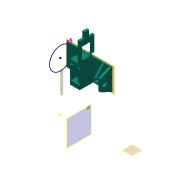
# Autodesk Inventor part: 30_Cube_XYZ_Stage_micrometer
Saved by Autodesk Inventor 2019 (Build 230136000, 136)
## iProperties
Created: 2020-01-27
Part Number: 30_Cube_XYZ_Stage_micrometer
Material: Generic
Document SubType Name: Modeling
Designer: diederichbenedict
Density: 1 g/cm^3
Appearance: IPHT_Türkis
Author: diederichbenedict
Autodesk Inventor part; units mm, degrees
ref_plane "Work Plane1" through (-87, 111.025, -16.9) normal (0, 0, 1) x (0, -1, 0)
ref_plane "Work Plane2" through (-77.1, 158.7453, 0.9792) normal (-1, 0, 0) x (0, 0, 1)
sketch "Sketch2" plane through (-77.1, 158.7453, 0.9792) normal (-1, 0, 0) x (0, 0, 1)
  circle A0 centre (-3.6792, 33.2797) radius 0.9 projected
  circle A1 centre (12.0208, -13.4394) radius 0.9 projected
  circle A2 centre (-14.9792, -12.5703) radius 0.9 projected
  line L0 (4.6208, 1.0297) -> (4.6208, 8.2797) projected
  line L1 (-4.8792, 8.2797) -> (-4.8792, 1.0297) projected
  line L2 (-4.8792, 1.0297) -> (4.6208, 1.0297) projected
  line L3 (4.6208, 8.2797) -> (-4.8792, 8.2797) projected
  line L4 (15.3208, -8.9703) -> (15.3208, 6.4797) projected
  line L5 (-5.6792, 35.2797) -> (3.4208, 35.2797) projected
  line L6 (20.1208, 22.4797) -> (4.1208, 22.4797) projected
  line L7 (-22.6852, 20.4797) -> (-8.6792, 20.4797) projected
  line L8 (15.3208, 6.4797) -> (15.3208, 22.4797)
  line L9 (15.3208, 22.4797) -> (4.1208, 22.4797)
  line L10 (4.1208, 22.4797) -> (4.1208, 35.2797)
  line L11 (4.1208, 35.2797) -> (-5.6792, 35.2797)
  line L12 (-16.3292, -14.4703) -> (-17.9792, -12.8203) projected
  line L13 (-16.3292, -14.4703) -> (-11.8329, -14.4703)
  line L14 (-11.8329, -14.4703) -> (-11.8329, -22.4688)
  line L15 (-11.8329, -22.4688) -> (15.3208, -22.4688)
  line L16 (15.3208, -22.4688) -> (15.3208, 6.4797)
  line L17 (9.9041, -17.695) -> (9.9041, 9.5842)
  line L18 (9.9041, 9.5842) -> (-12.605, 9.5842)
  line L19 (-12.605, 9.5842) -> (-12.605, -12.6165)
  line L20 (-12.605, -12.6165) -> (-10.7484, -12.6165)
  line L21 (-10.7484, -12.6165) -> (-5.6698, -17.695)
  line L22 (-5.6698, -17.695) -> (9.9041, -17.695)
  line L23 (-16.3292, -14.4703) -> (-17.8792, -12.9203)
  line L24 (-5.6792, 35.2797) -> (-5.6792, 20.4797)
  line L25 (-5.6792, 20.4797) -> (-17.8792, 20.4797)
  line L26 (-17.8792, -12.9203) -> (-17.8792, 20.4797)
  point P0 (-0.9792, -158.7453)
  constraints: 36 end point, 8 perpendicular, 3 collinear, 3 parallel, 3 vertical, 2 point on line, 1 horizontal
extrude "Extrusion1" add sketch "Sketch2" along normal blind 5 contours L16 L15 L14 L13 L12 L26 L7 L25 L24 L5 L11 L10 L6 L8 L4
sketch "Sketch3" plane through (-77.1, 158.7453, 0.9792) normal (1, 0, 0) x (0, -1, 0)
  circle A0 centre (-33.2797, 3.6792) radius 0.9 projected
  circle A1 centre (12.5703, 14.9792) radius 0.9 projected
  circle A2 centre (13.4394, -12.0208) radius 0.9 projected
  circle A3 centre (-33.2797, 3.6792) radius 2
  line L0 (-35.2797, -4.1208) -> (-35.2797, 5.6792) projected
  line L1 (14.4703, 16.3292) -> (14.4703, 11.8329) projected
  circle A4 centre (13.4394, -12.0208) radius 0.9 projected
  circle A5 centre (13.4394, -12.0208) radius 2
  circle A6 centre (12.5703, 14.9792) radius 1.9509
  point P0 (158.7453, 0.9792)
  dimension "d2" = 4
  constraints: 3 centre point, 3 coincident, 1 tangent
  measures "d2" diameter of A5
ref_plane "Work Plane6" through (-30.75, 17.2, 24.2) normal (0, -1, 0) x (1, 0, 0)
ref_plane "Work Plane8" through (-30.75, 12.2, 24.2) normal (0, -1, 0) x (1, 0, 0)
ref_plane "Work Plane3" through (-75, 13.4, 4.2) normal (0, -1, 0) x (1, 0, 0)
ref_plane "Work Plane7" through (-75, 18.4, 4.2) normal (0, -1, 0) x (1, 0, 0)
ref_plane "Work Plane9" through (-75, 13.4, 4.2) normal (0, -1, 0) x (1, 0, 0)
ref_plane "Work Plane4" through (-87, 111.025, -16.9) normal (0, 0, 1) x (0, -1, 0)
sketch "Sketch5" plane through (-87, 111.025, -16.9) normal (0, 0, 1) x (0, -1, 0)
  line L0 (-16.9, -46.4) -> (-16.9, -41.9) projected
  line L1 (-16.9, -41.9) -> (-21.4, -41.9) projected
  line L2 (-21.4, 41.9) -> (-21.4, -41.9) projected
  line L3 (-21.4, 41.9) -> (-16.9, 41.9) projected
  line L4 (-16.9, 41.9) -> (-16.9, 46.4) projected
  line L5 (-16.9, 46.4) -> (16.9, 46.4) projected
  line L6 (16.9, 46.4) -> (16.9, 41.9) projected
  line L7 (16.9, 41.9) -> (21.4, 41.9) projected
  line L8 (21.4, -41.9) -> (21.4, 41.9) projected
  line L9 (21.4, -41.9) -> (16.9, -41.9) projected
  line L10 (16.9, -41.9) -> (16.9, -46.4) projected
  line L11 (16.9, -46.4) -> (-16.9, -46.4) projected
  circle A0 centre (-19.9, 44.9) radius 1.45 projected
  circle A1 centre (-19.9, -44.9) radius 1.45 projected
  circle A2 centre (19.9, -44.9) radius 1.45 projected
  circle A3 centre (19.9, 44.9) radius 1.45 projected
  line L12 (-24.9, 47.9) -> (-24.9, -47.9) projected
  arc A4 (-24.9, -47.9) -> (-22.9, -49.9) centre (-22.9, -47.9) ccw projected
  line L13 (-22.9, -49.9) -> (22.9, -49.9) projected
  arc A5 (22.9, -49.9) -> (24.9, -47.9) centre (22.9, -47.9) ccw projected
  line L14 (24.9, -47.9) -> (24.9, 47.9) projected
  arc A6 (24.9, 47.9) -> (22.9, 49.9) centre (22.9, 47.9) ccw projected
  line L15 (22.9, 49.9) -> (-22.9, 49.9) projected
  arc A7 (-22.9, 49.9) -> (-24.9, 47.9) centre (-22.9, 47.9) ccw projected
  line L16 (-25.2515, 9.9) -> (-70.2, 9.9) projected
  line L17 (-24.9, 9.9) -> (24.9, 9.9)
  arc A8 (-19.2018, -3.8292) -> (-18.9105, -6.1599) centre (-19.9, -5.1) ccw
  arc A9 (-18.9105, 6.1599) -> (-19.2018, 3.8292) centre (-19.9, 5.1) ccw
  arc A10 (18.9105, -6.1599) -> (19.2018, -3.8292) centre (19.9, -5.1) ccw
  arc A11 (19.2018, 3.8292) -> (18.9105, 6.1599) centre (19.9, 5.1) ccw
  circle A12 centre (-19.9, -5.1) radius 1.45
  circle A13 centre (-19.9, 5.1) radius 1.45
  circle A14 centre (19.9, 5.1) radius 1.45
  circle A15 centre (19.9, -5.1) radius 1.45
  point P0 (111.025, 87)
  point P1 (-21.4, 9.9)
  point P2 (21.4, 9.9)
  constraints: 8 centre point, 8 point on circle, 7 point on line, 4 coincident, 4 concentric, 2 end point, 1 perpendicular, 16 other
ref_plane "Work Plane5" through (-136.9, 88.125, -16.9) normal (-1, 0, 0) x (0, 1, 0)
sketch "Sketch6" plane through (-136.9, 88.125, -16.9) normal (-1, 0, 0) x (0, 1, 0)
  line L0 (47.8, 0) -> (47.8, 6) projected
  line L1 (-2, 0) -> (-2, 6) projected
  line L2 (42.8, 8) -> (3, 8) projected
  circle A0 centre (22.9, -16.9) radius 24.9
  point P0 (-88.125, -16.9)
  constraints: 3 tangent, 1 centre point
extrude "Extrusion4" add sketch "Sketch5" along normal blind 3
sketch "Sketch7" plane through (-77.1, 181.225, 16.3) normal (0, 0, 1) x (0, -1, 0)
  line L0 (44.9485, 0) -> (0, 0) projected
  line L1 (0, 0) -> (0, -5) projected
  line L2 (44.9485, -5) -> (0, -5) projected
  line L3 (44.9485, 0) -> (44.9485, -5) projected
  circle A0 centre (90.1, -54.8) radius 1.45 projected
  circle A1 centre (50.3, -54.8) radius 1.45 projected
  line L4 (45.3, 38) -> (45.3, -57.8) projected
  arc A2 (45.3, -57.8) -> (47.3, -59.8) centre (47.3, -57.8) ccw projected
  line L5 (47.3, -59.8) -> (93.1, -59.8) projected
  arc A3 (93.1, -59.8) -> (95.1, -57.8) centre (93.1, -57.8) ccw projected
  line L6 (95.1, -57.8) -> (95.1, 38) projected
  line L7 (54.9485, 0) -> (54.9485, -0.5)
  line L8 (45.3, 38) -> (45.3, -57.8) projected
  line L9 (45.3, -5) -> (44.9485, -5)
  line L10 (54.9485, -22.1938) -> (54.9485, -21.6938)
  line L11 (54.9485, 0) -> (83.0578, 0)
  line L12 (83.0578, 0) -> (83.0578, -5)
  line L13 (83.0578, -5) -> (54.9485, -5)
  line L14 (54.9485, -5) -> (54.9485, 0)
  line L15 (54.9485, -22.1938) -> (83.0578, -22.1938)
  line L16 (83.0578, -22.1938) -> (83.0578, -17.1938)
  line L17 (83.0578, -17.1938) -> (54.9485, -17.1938)
  line L18 (54.9485, -17.1938) -> (54.9485, -22.1938)
  line L19 (83.0578, -22.1938) -> (86.0578, -22.1938)
  line L20 (86.0578, -22.1938) -> (86.0578, -21.6938)
  line L21 (86.0578, -21.6938) -> (83.0578, -21.6938)
  line L22 (83.0578, -21.6938) -> (83.0578, -22.1938)
  line L23 (83.0578, 0) -> (86.0578, 0)
  line L24 (86.0578, 0) -> (86.0578, -0.5)
  line L25 (86.0578, -0.5) -> (83.0578, -0.5)
  line L26 (83.0578, -0.5) -> (83.0578, 0)
  line L27 (95.1, -57.8) -> (95.1, 38) projected
  line L28 (86.0578, 0) -> (95.1, 0)
  line L29 (95.1, 0) -> (95.1, -22.1938)
  line L30 (95.1, -22.1938) -> (86.0578, -22.1938)
  line L31 (86.0578, -22.1938) -> (86.0578, 0)
  arc A4 (95.1, 38) -> (93.1, 40) centre (93.1, 38) ccw projected
  line L32 (93.1, 40) -> (47.3, 40) projected
  arc A5 (47.3, 40) -> (45.3, 38) centre (47.3, 38) ccw projected
  line L33 (44.9485, 0) -> (51.9485, 0)
  line L34 (51.9485, 0) -> (51.9485, -22.1938)
  line L35 (51.9485, -22.1938) -> (44.9485, -22.1938)
  line L36 (44.9485, -22.1938) -> (44.9485, 0)
  line L37 (51.9485, 0) -> (54.9485, 0)
  line L38 (54.9485, 0) -> (54.9485, -0.5)
  line L39 (54.9485, -0.5) -> (51.9485, -0.5)
  line L40 (51.9485, -0.5) -> (51.9485, 0)
  line L41 (51.9485, -22.1938) -> (54.9485, -22.1938)
  line L42 (54.9485, -22.1938) -> (54.9485, -21.6938)
  line L43 (54.9485, -21.6938) -> (51.9485, -21.6938)
  line L44 (51.9485, -21.6938) -> (51.9485, -22.1938)
  point P0 (181.225, 77.1)
  point P1 (37.3, 0)
  dimension "d10" = 0.5
  dimension "d12" = 0.5
  dimension "d13" = 5
  dimension "d14" = 3
  dimension "d15" = 0.5
  dimension "d37" = 3
  dimension "d40" = 7
  dimension "d41" = 3
  dimension "d42" = 0.5
  dimension "d43" = 3
  dimension "d44" = 0.5
  constraints: 70 end point, 16 parallel, 9 horizontal, 8 perpendicular, 6 point on line, 2 other
  measures "d10" distance of L7.start L7.end
  measures "d12" distance of L10.start L10.end
  measures "d13" distance of L16.end L15.end
  measures "d14" distance of L21.end L20.end
  measures "d15" distance of L20.end L19.end
  measures "d37" distance between parallel lines of L31 L12
  measures "d40" distance of L34.end L35.end
  measures "d41" distance of L38.end L39.end
  measures "d42" distance of L37.end L38.end
  measures "d43" distance of L43.end L42.end
  measures "d44" distance of L42.end L10.start
extrude "Extrusion5" add sketch "Sketch7" against normal blind 29 contours L33 L4 L9 L3 | L9 L4 L35 L36 | L33 L34 L35 L4 | L37 L7 L39 L34 | L11 L12 L13 L14 L7 | L34 L43 L10 L41 | L23 L24 L25 L12 | L10 L18 L17 L16 L15 | L28 L6 L30 L20 L31 L24 | L16 L21 L20 L19
sketch "Sketch8" plane through (-77.1, 181.225, -12.7) normal (0, 0, -1) x (0, 1, 0)
  line L0 (-95.1, 0) -> (-95.1, -22.1938) projected
  line L1 (-54.9485, -21.6938) -> (-54.9485, -17.1938) projected
  line L2 (-54.9485, -17.1938) -> (-83.0578, -17.1938) projected
  line L3 (-83.0578, -17.1938) -> (-83.0578, -21.6938) projected
  line L4 (-83.0578, -21.6938) -> (-86.0578, -21.6938) projected
  line L5 (-86.0578, -21.6938) -> (-86.0578, -0.5) projected
  line L6 (-86.0578, -0.5) -> (-83.0578, -0.5) projected
  line L7 (-83.0578, -0.5) -> (-83.0578, -5) projected
  line L8 (-83.0578, -5) -> (-54.9485, -5) projected
  line L9 (-54.9485, -5) -> (-54.9485, -0.5) projected
  line L10 (-44.9485, 0) -> (-95.1, 0) projected
  line L11 (-95.1, -22.1938) -> (-44.9485, -22.1938) projected
  line L12 (-44.9485, -22.1938) -> (-44.9485, 0) projected
  line L13 (-51.9485, -0.5) -> (-51.9485, -21.6938) projected
  line L14 (-51.9485, -21.6938) -> (-54.9485, -21.6938) projected
  line L15 (-54.9485, -0.5) -> (-51.9485, -0.5) projected
  line L16 (-95.1, -22.1938) -> (-86.0578, -22.1938)
  line L17 (-86.0578, -22.1938) -> (-86.0578, 0)
  line L18 (-86.0578, 0) -> (-95.1, 0)
  line L19 (-95.1, 0) -> (-95.1, -22.1938)
  constraints: 8 end point, 2 parallel, 1 horizontal, 1 perpendicular, 1 point on line
extrude "Extrusion6" add sketch "Sketch8" along normal up to surface (1.2 mm away) contours L10 L17 L5 L11 L0
sketch "Sketch9" plane through (-87, 111.025, -16.9) normal (0, 0, -1) x (0, 1, 0)
  circle A0 centre (-19.9, -5.1) radius 1.45 projected
  circle A1 centre (-19.9, 5.1) radius 1.45 projected
  point P0 (-111.025, 87)
extrude "Extrusion7" add sketch "Sketch9" against normal up to surface (33.2 mm away)
sketch "Sketch10" plane through (-37.1, 133.925, -16.9) normal (1, 0, 0) x (0, -1, 0)
  circle A0 centre (22.9, -16.9) radius 6.335 projected
  line L0 (35.4, -2.4) -> (35.4, -26.4) construction
  line L1 (35.4, -26.4) -> (10.4, -26.4) construction
  line L2 (10.4, -26.4) -> (10.4, -2.4) construction
  line L3 (10.4, -2.4) -> (35.4, -2.4) construction
  circle A1 centre (12.4, -4.4) radius 1.05 construction
  circle A2 centre (12.4, -16.9) radius 1.05 construction
  circle A3 centre (33.4, -16.9) radius 1.05 construction
  circle A4 centre (33.4, -4.4) radius 1.05 construction
  line L4 (17.4, -8) -> (14.4, -8) construction
  line L5 (17.4, -6) -> (17.4, -8) construction
  line L6 (14.4, -6) -> (17.4, -6) construction
  line L7 (14.4, -8) -> (14.4, -6) construction
  line L8 (47.8, 0) -> (47.8, 6) construction
  line L9 (-2, 0) -> (-2, 6) construction
  line L10 (47.8, 0) -> (35.4, -26.4)
  line L11 (35.4, -26.4) -> (10.4, -26.4)
  line L12 (10.4, -26.4) -> (-2, 0)
  line L13 (-2, 0) -> (47.8, 0)
  circle A5 centre (33.4, -4.4) radius 1.05 projected
  circle A6 centre (33.4, -16.9) radius 1.05 projected
  circle A7 centre (12.4, -4.4) radius 1.05 projected
  circle A8 centre (12.4, -16.9) radius 1.05 projected
  circle A9 centre (33.4, -4.4) radius 0.75
  circle A10 centre (33.4, -16.9) radius 0.75
  circle A11 centre (12.4, -4.4) radius 0.75
  circle A12 centre (12.4, -16.9) radius 0.75
  point P0 (133.925, -16.9)
  dimension "d45" = 1.5
  dimension "d46" = 1.5
  dimension "d47" = 1.5
  dimension "d48" = 1.5
  constraints: 8 end point, 4 centre point, 4 coincident, 1 collinear, 1 perpendicular
  measures "d45" diameter of A9
  measures "d46" diameter of A10
  measures "d47" diameter of A11
  measures "d48" diameter of A12
extrude "Extrusion8" add sketch "Sketch10" against normal blind 5 contours L10 L11 L12 L13
sketch "Sketch15" plane through (-42.1, 133.925, -16.9) normal (-1, 0, 0) x (0, -1, 0)
  circle A0 centre (33.4, 4.4) radius 1.05 projected
  circle A1 centre (33.4, 16.9) radius 1.05 projected
  circle A2 centre (12.4, 4.4) radius 1.05 projected
  circle A3 centre (12.4, 16.9) radius 1.05 projected
  line L0 (35.398, 2.4813) -> (31.4341, 2.4813)
  line L1 (31.4341, 2.4813) -> (31.4341, 18.8854)
  line L2 (31.4341, 18.8854) -> (35.398, 18.8854)
  line L3 (35.398, 18.8854) -> (35.398, 2.4813)
  line L4 (10.368, 2.4813) -> (14.0327, 2.4813)
  line L5 (14.0327, 2.4813) -> (14.0327, 18.5364)
  line L6 (14.0327, 18.5364) -> (10.368, 18.5364)
  line L7 (10.368, 18.5364) -> (10.368, 2.4813)
  point P0 (133.925, 16.9)
  constraints: 16 end point, 4 parallel, 2 horizontal, 2 perpendicular, 1 point on line
ref_plane "Work Plane14" through (8, -4.95, -16.9) normal (0, 1, 0) x (-1, 0, 0)
ref_plane "Work Plane15" through (-4.5, 41.5, 2.4) normal (0, 1, 0) x (0, 0, 1)
ref_plane "Work Plane19" through (-45.5, 98.525, -14.5) normal (1, 0, 0) x (0, 1, 0)
extrude "Extrusion16" add sketch "Sketch15" along normal up to surface (3.4 mm away)
sketch "Sketch18" plane through (-87, 111.025, -13.9) normal (0, 0, 1) x (0, -1, 0)
  line L0 (12.5, 40.6) -> (-12.5, 40.6) projected
  line L1 (12.5, 40.6) -> (-12.5, 40.6) projected
  line L2 (12.5, 41.5) -> (12.5, 40.6) projected
  line L3 (12.5, 41.5) -> (10.4, 41.5) projected
  line L4 (10.4, 43.9) -> (10.4, 41.5) projected
  line L5 (-10.4, 43.9) -> (10.4, 43.9) projected
  line L6 (-10.4, 43.9) -> (-10.4, 41.5) projected
  line L7 (-10.4, 41.5) -> (-12.5, 41.5) projected
  line L8 (-12.5, 41.5) -> (-12.5, 40.6) projected
  line L9 (8, 42.7) -> (8, 43.1) projected
  line L10 (-8, 42.7) -> (8, 42.7) projected
  line L11 (-8, 43.1) -> (-8, 42.7) projected
  line L12 (8, 43.1) -> (-8, 43.1) projected
  line L13 (-12.9725, 39.4492) -> (13.4306, 39.4492)
  line L14 (13.4306, 39.4492) -> (13.4306, 41.5)
  line L15 (13.4306, 41.5) -> (-12.9725, 41.5)
  line L16 (-12.9725, 41.5) -> (-12.9725, 39.4492)
  point P0 (111.025, 87)
  constraints: 8 end point, 2 parallel, 1 horizontal, 1 perpendicular
extrude "Extrusion17" cut sketch "Sketch18" against normal blind 10 contours L2 L15 L14 L13 L16 L8 L0 | L0 L8 L7 L15 L3 L2
ref_plane "Work Plane16" through (-56.9017, 111.025, 0) normal (-1, 0, 0) x (0, -1, 0)
sketch "Sketch19" plane through (-56.9017, 111.025, 0) normal (-1, 0, 0) x (0, -1, 0)
  line L0 (-4, 4) -> (-4, -4) projected
  line L1 (4, 4) -> (-4, 4) projected
  line L2 (4, -4) -> (4, 4) projected
  line L3 (3.85, -4.1) -> (-3.85, -4.1) projected
  line L4 (-4, -4) -> (4, -4) projected
  line L5 (-4.2, 4.2) -> (-4.2, -4.2)
  line L6 (-4.2, -4.2) -> (4.2, -4.2)
  line L7 (4.2, -4.2) -> (4.2, 4.2)
  line L8 (4.2, 4.2) -> (-4.2, 4.2)
  line L9 (-4.2, 4.2) -> (-24.782, -13.9028)
  line L10 (-24.782, -13.9028) -> (24.8985, -13.9028)
  line L11 (24.8985, -13.9028) -> (4.2, 4.2)
  circle A0 centre (-7.6854, -9.3896) radius 1.2208
  point P0 (111.025, 0)
  dimension "d60" = 0.2
  constraints: 14 end point, 1 centre point, 1 horizontal, 3 other
  measures "d60" distance between parallel lines of L1 L8
ref_plane "Work Plane17" through (4.15, 35.0983, 12.8) normal (0, 1, 0) x (0, 0, 1)
ref_plane "Work Plane18" through (-51.9017, 107.175, -4.1) normal (1, 0, 0) x (0, 1, 0)
extrude "Extrusion18" add sketch "Sketch19" against normal up to surface (5 mm away) contours L5 L6 L7 L11 L10 L9
sketch "Sketch20" plane through (-77.1, 158.7453, 0.9792) normal (1, 0, 0) x (0, 0, -1)
  circle A0 centre (3.6792, 33.2797) radius 0.9 projected
  line L0 (9.9704, -2.9576) -> (-8.0296, -2.9576) projected
  line L1 (-8.0296, -2.9576) -> (-8.0296, 11.8541) projected
  line L2 (-8.0296, 11.8541) -> (9.9674, 11.8541) projected
  arc A1 (9.9704, 11.8244) -> (9.9674, 11.8541) centre (12.8292, 12.1297) ccw projected
  line L3 (9.9704, 11.8244) -> (9.9704, -2.9576) projected
  circle A2 centre (-7.8502, -6.7996) radius 2.875 projected
  line L4 (-11.4796, 8.9797) -> (-11.4796, -53.7279) projected
  line L5 (13.4189, -53.7279) -> (-11.4796, -53.7279) projected
  line L6 (13.4189, -13.7279) -> (13.4189, -53.7279) projected
  line L7 (13.4189, -13.7279) -> (21.5204, -13.7279) projected
  line L8 (21.5204, -13.7279) -> (21.5204, 26.2721) projected
  line L9 (21.5204, 26.2721) -> (-11.4796, 26.2721) projected
  line L10 (-11.4796, 26.2721) -> (-11.4796, 11.2944) projected
  line L11 (-11.4796, 11.2944) -> (-11.5208, 11.2531) projected
  line L12 (-11.5208, 11.2531) -> (-11.5208, 8.9797) projected
  line L13 (-11.5208, 8.9797) -> (-11.4796, 8.9797) projected
  circle A3 centre (14.9792, -12.5703) radius 0.9 projected
  circle A4 centre (-12.0208, -13.4394) radius 0.9 projected
  circle A5 centre (14.9792, -12.5703) radius 2
  circle A6 centre (-12.0208, -13.4394) radius 2
  circle A7 centre (3.6792, 33.2797) radius 2
  point P0 (0.9792, -158.7453)
  dimension "d63" = 4
  dimension "d64" = 4
  dimension "d65" = 4
  constraints: 3 centre point, 3 coincident
  measures "d63" diameter of A5
  measures "d64" diameter of A6
  measures "d65" diameter of A7
ref_plane "Work Plane20" through (-74.5, 162.725, -23.9) normal (-1, 0, 0) x (0, 0, 1)
extrude "Extrusion19" add sketch "Sketch20" along normal up to surface (2.6 mm away) contours A6 L4 A4 | L4 A4 A6 | A5 L7 L6 | L6 L7 A5 | A7
sketch "Sketch21" plane through (-74.5, 192.025, -2.7) normal (1, 0, 0) x (0, 0, -1)
  circle A0 centre (0, 0) radius 0.9 projected
  line L0 (-7.1, -0.5) -> (-7.1, 2) projected
  line L1 (-5.6, -0.5) -> (-7.1, -0.5) projected
  line L2 (-5.6, -2) -> (-5.6, -0.5) projected
  line L3 (2, -2) -> (-5.6, -2) projected
  line L4 (2, 2) -> (2, -2) projected
  line L5 (-7.1, 2) -> (2, 2) projected
  circle A1 centre (0, 0) radius 2 projected
  circle A2 centre (0, 0) radius 0.9 projected
  point P0 (-2.7, -192.025)
ref_plane "Work Plane21" through (-73.6, 179.225, -12.7) normal (-1, 0, 0) x (0, 0, 1)
extrude "Extrusion20" add sketch "Sketch21" along normal up to surface (0.9 mm away) contours A1
sketch "Sketch22" plane through (-87, 111.025, -13.9) normal (0, 0, 1) x (1, 0, 0)
  line L0 (35.0983, -24.8953) -> (30.0983, -24.8953) projected
  line L1 (30.0983, -24.8953) -> (30.0983, 24.7788) projected
  line L2 (30.0983, 24.7788) -> (35.0983, 24.7788) projected
  line L3 (35.0983, 24.7788) -> (35.0983, -24.8953) projected
  circle A0 centre (5.1, 19.9) radius 1.45 projected
  circle A1 centre (-5.1, 19.9) radius 1.45 projected
  circle A2 centre (-44.9, -19.9) radius 1.45 projected
  circle A3 centre (-44.9, 19.9) radius 1.45 projected
  line L4 (41.5, -12.498) -> (41.5, -13.4306) projected
  line L5 (41.5, -13.4306) -> (39.4492, -13.4306) projected
  line L6 (39.4492, -13.4306) -> (39.4492, 12.9725) projected
  line L7 (39.4492, 12.9725) -> (41.5, 12.9725) projected
  line L8 (41.5, 12.9725) -> (41.5, 12.532) projected
  line L9 (41.5, 12.532) -> (44.9, 12.532) projected
  line L10 (44.9, 12.532) -> (44.9, 18.45) projected
  arc A4 (44.9, 21.35) -> (44.9, 18.45) centre (44.9, 19.9) ccw projected
  line L11 (44.9, 21.35) -> (44.9, 23.4909) projected
  line L12 (44.9, 23.4909) -> (49.8107, 23.4909) projected
  arc A5 (49.8107, 23.4909) -> (47.9, 24.9) centre (47.9, 22.9) ccw projected
  line L13 (47.9, 24.9) -> (-47.9, 24.9) projected
  arc A6 (-47.9, 24.9) -> (-49.9, 22.9) centre (-47.9, 22.9) ccw projected
  line L14 (-49.9, 22.9) -> (-49.9, -22.9) projected
  arc A7 (-49.9, -22.9) -> (-47.9, -24.9) centre (-47.9, -22.9) ccw projected
  line L15 (-47.9, -24.9) -> (-12.2938, -24.9) projected
  line L16 (-12.2938, -24.9) -> (-12.2938, -15.8578) projected
  line L17 (-12.2938, -15.8578) -> (9.9, -15.8578) projected
  line L18 (9.9, -15.8578) -> (9.9, -24.9) projected
  line L19 (9.9, -24.9) -> (47.9, -24.9) projected
  arc A8 (47.9, -24.9) -> (49.8107, -23.4909) centre (47.9, -22.9) ccw projected
  line L20 (49.8107, -23.4909) -> (44.9, -23.4909) projected
  line L21 (44.9, -23.4909) -> (44.9, -21.35) projected
  arc A9 (44.9, -18.45) -> (44.9, -21.35) centre (44.9, -19.9) ccw projected
  line L22 (44.9, -18.45) -> (44.9, -12.498) projected
  line L23 (44.9, -12.498) -> (41.5, -12.498) projected
  line L24 (-18.4513, 24.9) -> (-23.4513, 24.9)
  line L25 (-23.4513, 24.9) -> (-23.4513, 0)
  line L26 (-23.4513, 0) -> (-18.4513, 0)
  line L27 (-18.4513, 0) -> (-18.4513, 24.9)
  line L28 (-49.9, 22.9) -> (-49.9, -22.9) projected
  line L29 (-23.4513, 24.9) -> (-49.9, 24.9)
  line L30 (-49.9, 24.9) -> (-49.9, 17.9)
  line L31 (-49.9, 17.9) -> (-23.4513, 17.9)
  line L32 (-23.4513, 17.9) -> (-23.4513, 24.9)
  point P0 (87, -111.025)
  dimension "d70" = 5
  dimension "d71" = 24.9
  dimension "d72" = 7
  constraints: 16 end point, 4 parallel, 2 horizontal, 2 perpendicular, 2 point on line
  measures "d70" distance of L26.end L25.end
  measures "d71" distance of L25.end L24.end
  measures "d72" distance of L30.end L29.end
extrude "Extrusion21" add sketch "Sketch22" along normal blind 15 contours L27 L26 L25 L13 | L25 L31 L14 A6 L13 | A6 L30 L29
sketch "Sketch23" plane through (-110.4513, 111.025, -13.9) normal (-1, 0, 0) x (0, 0, 1)
  line L0 (15, 17.9) -> (0, 17.9) projected
  line L1 (0, 0) -> (0, 17.9) projected
  line L2 (0, 0) -> (15, 0) projected
  line L3 (15, 17.9) -> (15, 0) projected
  circle A0 centre (11.1856, 4.9118) radius 1.4
  point P0 (13.9, -111.025)
  dimension "d75" = 2.8
  constraints: 1 centre point
  measures "d75" diameter of A0
extrude "Extrusion22" cut sketch "Sketch23" against normal up to surface (11.1575 mm away) contours A0
fillet "Fillet2" radius 2 3 edges at (-107.9513, 111.025, 1.1) (-107.9513, 111.025, -13.9) (-110.4513, 128.925, -6.4)
body "Solid1"
